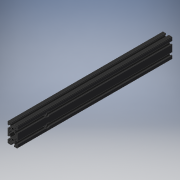
# Autodesk Inventor part: HFS5-2040-320-TPW-Z5-YA62.5
Saved by Autodesk Inventor 2019 (Build 230136000, 136)
## iProperties
Created: 2022-12-16
Part Number: HFS5-2040-320-TPW-Z5-YA62.5
Material: Generic
Catalog Web Link: www.cadenas.de
Description: NFS5-2040, NFSB5-2040, HFS5-2040, HFSB5-2040, CAF5-2040, NFSF5-2040, HFSF5-2040, HFSY5-2040-Aluminum Frames -5 Series-2Row Groove 20x40 mm Square -Specified Length
Vendor: MISUMI
Document SubType Name: Modeling
Designer: psAdmin
Manufacturer: MISUMI
Mass: 103.283 g
Surface Area: 1011.21 cm^2
Volume: 103.283 cm^3
Density: 1 g/cm^3
Appearance: PSOLRGB-175-175-175
Category: PARTsolutions
Company: MISUMI
Title: HFS5-2040-320-TPW-Z5-YA62.5
Author: Cadenas PARTsolutions
Comments: Aluminum Frames -5 Series-2Row Groove 20x40 mm Square -Specified Length
PSOL_IDENT_0: {$CADENAS_DATA/23d-libs/misumi/metric/38_al_extrusions_blackets/5/hfs5_2040.prj},655 {VTYP=3D},{NB=H
PSOL_IDENT_1: FS5-2040-320-TPW-Z5-YA62.5},{LINA=HFS5-2040-320-TPW-Z5-YA62.5},{NN=NFS5-2040, NFSB5-2040, HFS5-2040,
PSOL_IDENT_2: HFSB5-2040, CAF5-2040, NFSF5-2040, HFSF5-2040, HFSY5-2040},{DATE=23.09.2021 05:44:57},{GEOMDATE=23.
PSOL_IDENT_3: 09.2021 02:57:03},{VERSION=},{LINEID=150},{WBVAR=L,ALT1,ALT2,ALT4,ALT5,CP5,DL5,DR5,ALT6,ALT9,ALT10,A
PSOL_IDENT_4: LT11,HP6,NHL6,DL6,NHR6,DR6,ALT7,ALT8,NH9,AH,BH,CH,DH,EH,NH10,AV,BV,CV,DV,EV,NH11,AP,BP,CP,DP,EP,ALT1
PSOL_IDENT_5: 2,ALT13,Z,NH12,XA,XB,XC,XD,XE,NH13,YA,YB,YC,YD,YE,ALT16,HP16,DL16,DR16,ALT17,HQ17,JLP,ALT18,HQ18,KLP
PSOL_IDENT_6: ,ALT20},{WBNUMERIC=L,NH9,AH,BH,CH,DH,EH,NH10,AV,BV,CV,DV,EV,NH11,AP,BP,CP,DP,EP,NH12,XA,XB,XC,XD,XE,
PSOL_IDENT_7: NH13,YA,YB,YC,YD,YE,HQ17,JLP,HQ18,KLP}  {NB=HFS5-2040-320-TPW-Z5-YA62.5},{LINA=HFS5-2040-320-TPW-Z5-
PSOL_IDENT_8: YA62.5},{KT=DUMMY},{PN=HFS5-2040-320-TPW-Z5-YA62.5},{TPS=HFS5-2040},{MAT=A6N01SS-T5 Aluminum Alloy},
PSOL_IDENT_9: {ST=Clear Anodize},{FRMW=20},{FRMH=40},{FRD=4.2},{L=320},{MASS=0.88},{SA=324},{LX=1.358x10^4},{LY=5.
PSOL_IDENT_10: 13x10^4},{ALT1=TPW},{M1=5},{DPL1=15},{DPR1=15},{ALT1PN=-TPW},{ALT2=},{ALT2ALG= '','Not applicable' }
PSOL_IDENT_11: ,{M2=0},{DP2=0},{ALT2PN=},{ALT4=},{ALT4ALG= '', 'w/o SC (High Precision Cut)', 'SC', 'with SC (High
PSOL_IDENT_12: Precision Cut)' },{ALT4PN=},{ALT5=},{ALT5ALG= '','w/o 45 Degree Cut','1','with 45 Degree Cut' },{CP5=
PSOL_IDENT_13: },{CP5ALG= '','N/A' },{DL5=},{DL5ALG= '','N/A' },{DR5=},{DR5ALG= '','N/A' },{FRMLALT5=0},{FRMRALT5=0
PSOL_IDENT_14: },{ALT5PN=},{ALT6=},{ALT6ALG= '','w/o Fastening Location Wrench Access Hole Alterations','1','with F
PSOL_IDENT_15: astening Location Wrench Access Hole Alterations' },{ALT9=},{ALT9ALG= '','w/o Location Specified Wre
PSOL_IDENT_16: nch Access Hole Alteratons (Horizontal)','1','with Location Specified Wrench Access Hole Alteratons
PSOL_IDENT_17: (Horizontal)' },{ALT10=},{ALT10ALG= '','w/o Location Specified Wrench Access Hole Alteratons (Vertic
PSOL_IDENT_18: al)','1','with Location Specified Wrench Access Hole Alteratons (Vertical)' },{ALT11=},{ALT11ALG= ''
PSOL_IDENT_19: ,'w/o Location Specified Wrench Access Hole Alteratons (Crisscross)','1','with Location Specified Wr
PSOL_IDENT_20: ench Access Hole Alteratons (Crisscross)' },{HP6=},{HP6ALG= '','N/A' },{NHL6=},{NHL6ALG= '','N/A' },
PSOL_IDENT_21: {DL6=},{DL6ALG= '','N/A' },{NHR6=},{NHR6ALG= '','N/A' },{DR6=},{DR6ALG= '','N/A' },{HL6=0},{HL6D=0},
PSOL_IDENT_22: {HR6=0},{HR6D=0},{J6=0},{J6D=0},{K6=0},{K6D=0},{DD6=0.00},{DD6ALG=0},{ALT7=},{ALT7ALG= '','N/A' },{A
PSOL_IDENT_23: LT8=},{ALT8ALG= '','N/A' },{ALT678PN=},{NH9=0},{NH9MAX=5},{NH9ALG=[0]},{AH=0.0},{AHMIN=7},{AHMAX=315
PSOL_IDENT_24: },{AHALG=[0]},{BH=0.0},{BHMIN=2},{BHMAX=317},{BHALG=[0]},{CH=0.0},{CHMIN=2},{CHMAX=319},{CHALG=[0]},
PSOL_IDENT_25: {DH=0.0},{DHMIN=2},{DHMAX=321},{DHALG=[0]},{EH=0.0},{EHMIN=2},{EHMAX=313},{EHALG=[0]},{NH10=0},{NH10
PSOL_IDENT_26: MAX=5},{NH10ALG=[0]},{AV=0.0},{AVMIN=7},{AVMAX=315},{AVALG=[0]},{BV=0.0},{BVMIN=2},{BVMAX=317},{BVAL
PSOL_IDENT_27: G=[0]},{CV=0.0},{CVMIN=2},{CVMAX=319},{CVALG=[0]},{DV=0.0},{DVMIN=2},{DVMAX=321},{DVALG=[0]},{EV=0.0
PSOL_IDENT_28: },{EVMIN=2},{EVMAX=313},{EVALG=[0]},{NH11=0},{NH11MAX=5},{NH11ALG=[0]},{AP=0.0},{APMIN=7},{APMAX=315
PSOL_IDENT_29: },{APALG=[0]},{BP=0.0},{BPMIN=2},{BPMAX=317},{BPALG=[0]},{CP=0.0},{CPMIN=2},{CPMAX=319},{CPALG=[0]},
PSOL_IDENT_30: {DP=0.0},{DPMIN=2},{DPMAX=321},{DPALG=[0]},{EP=0.0},{EPMIN=2},{EPMAX=313},{EPALG=[0]},{ALT9PN=},{ALT
PSOL_IDENT_31: 10PN=},{ALT11PN=},{ALT91011PN=},{ALT12=},{ALT12ALG= '','w/o Counterbore Hole in Specified Position (
PSOL_IDENT_32: Vertical)','1','with Counterbore Hole in Specified Position (Vertical)' },{ALT13=1},{ALT13ALG= '','w
PSOL_IDENT_33: /o Counterbore Hole in Specified Position (Horizontal)','1','with Counterbore Hole in Specified Posi
PSOL_IDENT_34: tion (Horizontal)' },{Z=5},{ZALG='5','5','6','6'},{DD12=5.5},{DD112=9.5},{NH12=0},{NH12MAX=5},{NH12A
PSOL_IDENT_35: LG=[0]},{XA=0.0},{XAMIN=7},{XAMAX=324.5},{XAALG=[0]},{XB=0.0},{XBMIN=11.5},{XBMAX=336},{XBALG=[0]},{
PSOL_IDENT_36: XC=0.0},{XCMIN=11.5},{XCMAX=347.5},{XCALG=[0]},{XD=0.0},{XDMIN=11.5},{XDMAX=359},{XDALG=[0]},{XE=0.0
PSOL_IDENT_37: },{XEMIN=11.5},{XEMAX=313},{XEALG=[0]},{NH13=1},{NH13MAX=5},{NH13ALG=[1:5/1]},{YA=62.5},{YAMIN=7},{Y
PSOL_IDENT_38: AMAX=313},{YAALG=[7:313/0.5]},{YB=0.0},{YBMIN=74},{YBMAX=324.5},{YBALG=[0]},{YC=0.0},{YCMIN=11.5},{Y
PSOL_IDENT_39: CMAX=336},{YCALG=[0]},{YD=0.0},{YDMIN=11.5},{YDMAX=347.5},{YDALG=[0]},{YE=0.0},{YEMIN=11.5},{YEMAX=3
PSOL_IDENT_40: 13},{YEALG=[0]},{ALT12PN=},{ALT13PN=-YA62.5},{ALT1213PN=-Z5-YA62.5},{ALT16=},{ALT16ALG= '','w/o M Ty
PSOL_IDENT_41: pe Hole Alteration','1','with M Type Hole Alteration' },{HP16=},{HP16ALG= '','N/A' },{DL16=},{DL16AL
PSOL_IDENT_42: G= '','N/A' },{DR16=},{DR16ALG= '','N/A' },{H116=0},{D16=0.0},{ALT16PN=},{ALT17=},{ALT17ALG= '','w/o
PSOL_IDENT_43: L Type Hole Alteration (Top)','1','with L Type Hole Alteration (Top)' },{HQ17=0},{HQ17ALG=0},{JLP=0
PSOL_IDENT_44: },{JLPMIN=4.9},{JLPMAX=0},{JLPALG=[0]},{L17=0},{D17=0.0},{ALT18=},{ALT18ALG= '','w/o L Type Hole Alt
PSOL_IDENT_45: eration (Bottom)','1','with L Type Hole Alteration (Bottom)' },{HQ18=0},{HQ18ALG=0},{KLP=0},{KLPMIN=
PSOL_IDENT_46: 4.9},{KLPMAX=0},{KLPALG=[0]},{L18=0},{D18=0.0},{ALT1718PN=},{ALT20=},{ALT20PN=},{ERRORALT01=OK},{ERR
PSOL_IDENT_47: ORALT02=OK},{ERRORALT05=OK},{ERRORALT06091=OK},{ERRORALT06092=OK},{ERRORALT06093=OK},{ERRORALT06094=
PSOL_IDENT_48: OK},{ERRORALT06101=OK},{ERRORALT06102=OK},{ERRORALT06103=OK},{ERRORALT06104=OK},{ERRORALT06111=OK},{
PSOL_IDENT_49: ERRORALT06112=OK},{ERRORALT06113=OK},{ERRORALT06114=OK},{ERRORALT06121=OK},{ERRORALT06122=OK},{ERROR
PSOL_IDENT_50: ALT06123=OK},{ERRORALT06124=OK},{ERRORALT06131=OK},{ERRORALT06132=OK},{ERRORALT06133=OK},{ERRORALT06
PSOL_IDENT_51: 134=OK},{ERRORALT0616=OK},{ERRORALT06171=OK},{ERRORALT06172=OK},{ERRORALT06173=OK},{ERRORALT06181=OK
PSOL_IDENT_52: },{ERRORALT06182=OK},{ERRORALT06183=OK},{ERRORALT0911=OK},{ERRORALT0913=OK},{ERRORALT0916=OK},{ERROR
PSOL_IDENT_53: ALT0917=OK},{ERRORALT0918=OK},{ERRORALT1011=OK},{ERRORALT1012=OK},{ERRORALT1016=OK},{ERRORALT1017=OK
PSOL_IDENT_54: },{ERRORALT1018=OK},{ERRORALT1112=OK},{ERRORALT1113=OK},{ERRORALT1116=OK},{ERRORALT1117=OK},{ERRORAL
PSOL_IDENT_55: T1118=OK},{ERRORALT1216=OK},{ERRORALT1217=OK},{ERRORALT1218=OK},{ERRORALT1316=OK},{ERRORALT1317=OK},
PSOL_IDENT_56: {ERRORALT1318=OK},{ERRORALT1617=OK},{ERRORALT1618=OK},{ERRORPN=},{TFW=0},{COLOR=}
NB: HFS5-2040-320-TPW-Z5-YA62.5
NN: NFS5-2040, NFSB5-2040, HFS5-2040, HFSB5-2040, CAF5-2040, NFSF5-2040, HFSF5-2040, HFSY5-2040
NT: Aluminum Frames -5 Series-2Row Groove 20x40 mm Square -Specified Length
NBSYN: $PN.
LINA: HFS5-2040-320-TPW-Z5-YA62.5
CATALOG: Misumi
PN: HFS5-2040-320-TPW-Z5-YA62.5
TPS: HFS5-2040
MAT: A6N01SS-T5 Aluminum Alloy
ST: Clear Anodize
L: 320
MASS: 0.88
SA: 324
LX: 1.358x10^4
LY: 5.13x10^4
ALT1: with TPW (Tapping on Both Ends)
M1: 5
DPL1: 15
DPR1: 15
ALT2: Not applicable
M2: 0
DP2: 0
ALT4: w/o SC (High Precision Cut)
ALT5: w/o 45 Degree Cut
CP5: N/A
DL5: N/A
DR5: N/A
ALT6: w/o Fastening Location Wrench Access Hole Alterations
ALT9: w/o Location Specified Wrench Access Hole Alteratons (Horizontal)
ALT10: w/o Location Specified Wrench Access Hole Alteratons (Vertical)
ALT11: w/o Location Specified Wrench Access Hole Alteratons (Crisscross)
HP6: N/A
NHL6: N/A
DL6: N/A
NHR6: N/A
DR6: N/A
HL6D: 0
HR6D: 0
J6D: 0
K6D: 0
DD6: 0
ALT7: N/A
ALT8: N/A
NH9: 0
AH: 0
BH: 0
CH: 0
DH: 0
EH: 0
NH10: 0
AV: 0
BV: 0
CV: 0
DV: 0
EV: 0
NH11: 0
AP: 0
BP: 0
CP: 0
DP: 0
EP: 0
ALT12: w/o Counterbore Hole in Specified Position (Vertical)
ALT13: with Counterbore Hole in Specified Position (Horizontal)
Z: 5
DD12: 5.5
DD112: 9.5
NH12: 0
XA: 0
XB: 0
XC: 0
XD: 0
XE: 0
NH13: 1
YA: 62.5
YB: 0
YC: 0
YD: 0
YE: 0
ALT16: w/o M Type Hole Alteration
HP16: N/A
DL16: N/A
DR16: N/A
H116: 0
D16: 0
ALT17: w/o L Type Hole Alteration (Top)
HQ17: 0
JLP: 0
D17: 0
ALT18: w/o L Type Hole Alteration (Bottom)
HQ18: 0
KLP: 0
D18: 0
ALT20: w/o CW (End Face C Chamfering)
SUPPLIER: MISUMI
ARTICLENO: HFS5-2040-320-TPW-Z5-YA62.5
BOMINFO: HFS5-2040-320-TPW-Z5-YA62.5
CREATOR: CADENAS GmbH
Autodesk Inventor part; units mm, degrees
ref_plane "YZ Plane" through (0, 0, 0) normal (1, 0, 0) x (0, 1, 0)
ref_plane "XZ Plane" through (0, 0, 0) normal (0, 1, 0) x (-1, 0, 0)
ref_plane "XY Plane" through (0, 0, 0) normal (0, 0, 1) x (1, 0, 0)
sketch "Sketch_1" plane through (0, 0, 0) normal (0, 0, 1) x (1, 0, 0)
  line L0 (-10, -7) -> (-8, -7)
  line L1 (-8, -7) -> (-8, -4)
  line L2 (-8, -4) -> (-7.0607, -4)
  line L3 (-7.0607, -4) -> (-4, -7.0607)
  line L4 (-4, -7.0607) -> (-4, -9.4804)
  line L5 (-4, -9.4804) -> (-3.7, -10)
  line L6 (-3.7, -10) -> (-4, -10.5196)
  line L7 (-4, -10.5196) -> (-4, -12.9393)
  line L8 (-4, -12.9393) -> (-7.0607, -16)
  line L9 (-7.0607, -16) -> (-8, -16)
  line L10 (-8, -16) -> (-8, -13)
  line L11 (-8, -13) -> (-10, -13)
  line L12 (-10, -13) -> (-10, -19)
  arc A0 (-10, -19) -> (-9, -20) centre (-9, -19) ccw
  line L13 (-9, -20) -> (-3, -20)
  line L14 (-3, -20) -> (-3, -18)
  line L15 (-3, -18) -> (-6, -18)
  line L16 (-6, -18) -> (-6, -17.0607)
  line L17 (-6, -17.0607) -> (-2.9393, -14)
  line L18 (-2.9393, -14) -> (-0.5196, -14)
  line L19 (-0.5196, -14) -> (0, -13.7)
  line L20 (0, -13.7) -> (0.5196, -14)
  line L21 (0.5196, -14) -> (2.9393, -14)
  line L22 (2.9393, -14) -> (6, -17.0607)
  line L23 (6, -17.0607) -> (6, -18)
  line L24 (6, -18) -> (3, -18)
  line L25 (3, -18) -> (3, -20)
  line L26 (3, -20) -> (9, -20)
  arc A1 (9, -20) -> (10, -19) centre (9, -19) ccw
  line L27 (10, -19) -> (10, -13)
  line L28 (10, -13) -> (8, -13)
  line L29 (8, -13) -> (8, -16)
  line L30 (8, -16) -> (7.0607, -16)
  line L31 (7.0607, -16) -> (4, -12.9393)
  line L32 (4, -12.9393) -> (4, -10.5196)
  line L33 (4, -10.5196) -> (3.7, -10)
  line L34 (3.7, -10) -> (4, -9.4804)
  line L35 (4, -9.4804) -> (4, -7.0607)
  line L36 (4, -7.0607) -> (7.0607, -4)
  line L37 (7.0607, -4) -> (8, -4)
  line L38 (8, -4) -> (8, -7)
  line L39 (8, -7) -> (10, -7)
  line L40 (10, -7) -> (10, 7)
  line L41 (10, 7) -> (8, 7)
  line L42 (8, 7) -> (8, 4)
  line L43 (8, 4) -> (7.0607, 4)
  line L44 (7.0607, 4) -> (4, 7.0607)
  line L45 (4, 7.0607) -> (4, 9.4804)
  line L46 (4, 9.4804) -> (3.7, 10)
  line L47 (3.7, 10) -> (4, 10.5196)
  line L48 (4, 10.5196) -> (4, 12.9393)
  line L49 (4, 12.9393) -> (7.0607, 16)
  line L50 (7.0607, 16) -> (8, 16)
  line L51 (8, 16) -> (8, 13)
  line L52 (8, 13) -> (10, 13)
  line L53 (10, 13) -> (10, 19)
  arc A2 (10, 19) -> (9, 20) centre (9, 19) ccw
  line L54 (9, 20) -> (3, 20)
  line L55 (3, 20) -> (3, 18)
  line L56 (3, 18) -> (6, 18)
  line L57 (6, 18) -> (6, 17.0607)
  line L58 (6, 17.0607) -> (2.9393, 14)
  line L59 (2.9393, 14) -> (0.5196, 14)
  line L60 (0.5196, 14) -> (0, 13.7)
  line L61 (0, 13.7) -> (-0.5196, 14)
  line L62 (-0.5196, 14) -> (-2.9393, 14)
  line L63 (-2.9393, 14) -> (-6, 17.0607)
  line L64 (-6, 17.0607) -> (-6, 18)
  line L65 (-6, 18) -> (-3, 18)
  line L66 (-3, 18) -> (-3, 20)
  line L67 (-3, 20) -> (-9, 20)
  arc A3 (-9, 20) -> (-10, 19) centre (-9, 19) ccw
  line L68 (-10, 19) -> (-10, 13)
  line L69 (-10, 13) -> (-8, 13)
  line L70 (-8, 13) -> (-8, 16)
  line L71 (-8, 16) -> (-7.0607, 16)
  line L72 (-7.0607, 16) -> (-4, 12.9393)
  line L73 (-4, 12.9393) -> (-4, 10.5196)
  line L74 (-4, 10.5196) -> (-3.7, 10)
  line L75 (-3.7, 10) -> (-4, 9.4804)
  line L76 (-4, 9.4804) -> (-4, 7.0607)
  line L77 (-4, 7.0607) -> (-7.0607, 4)
  line L78 (-7.0607, 4) -> (-8, 4)
  line L79 (-8, 4) -> (-8, 7)
  line L80 (-8, 7) -> (-10, 7)
  line L81 (-10, 7) -> (-10, -7)
  line L82 (-8, 1.7) -> (-8, -1.7)
  arc A4 (-8, -1.7) -> (-7.7, -2) centre (-7.7, -1.7) ccw
  line L83 (-7.7, -2) -> (-7.0636, -2)
  arc A5 (-6.8515, -2.0879) -> (-7.0636, -2) centre (-7.0636, -2.3) ccw
  line L84 (-6.8515, -2.0879) -> (-2.9393, -6)
  line L85 (-2.9393, -6) -> (2.9393, -6)
  line L86 (2.9393, -6) -> (6.8515, -2.0879)
  arc A6 (7.0636, -2) -> (6.8515, -2.0879) centre (7.0636, -2.3) ccw
  line L87 (7.0636, -2) -> (7.7, -2)
  arc A7 (7.7, -2) -> (8, -1.7) centre (7.7, -1.7) ccw
  line L88 (8, -1.7) -> (8, 1.7)
  arc A8 (8, 1.7) -> (7.7, 2) centre (7.7, 1.7) ccw
  line L89 (7.7, 2) -> (7.0636, 2)
  arc A9 (6.8515, 2.0879) -> (7.0636, 2) centre (7.0636, 2.3) ccw
  line L90 (6.8515, 2.0879) -> (2.9393, 6)
  line L91 (2.9393, 6) -> (-2.9393, 6)
  line L92 (-2.9393, 6) -> (-6.8515, 2.0879)
  arc A10 (-7.0636, 2) -> (-6.8515, 2.0879) centre (-7.0636, 2.3) ccw
  line L93 (-7.0636, 2) -> (-7.7, 2)
  arc A11 (-7.7, 2) -> (-8, 1.7) centre (-7.7, 1.7) ccw
  constraints: 188 end point, 24 point on circle, 12 centre point
extrude "Extrusion1" add sketch "Sketch_1" against normal blind 320
sketch "Sketch2" plane through (0, 0, 0) normal (0, 0, 1) x (1, 0, 0)
  point P0 (0, 10)
hole "Hole1" at (0, 10, 0) direction (0, 0, -1) diameter 4.134 depth 15 countersink diameter 5 countersink angle 90 thread size "M5x0.8" class "6H" standard "ISO Metric profile"
pattern_linear "Rectangular Pattern1" count 2 spacing 20 along (0, -1, 0) of "Hole1"
sketch "Sketch3" plane through (0, 0, -320) normal (0, 0, -1) x (-1, 0, 0)
  point P0 (0, 10)
hole "Hole2" at (0, 10, -320) direction (0, 0, 1) diameter 4.134 depth 15 countersink diameter 5 countersink angle 90 thread size "M5x0.8" class "6H" standard "ISO Metric profile"
pattern_linear "Rectangular Pattern2" count 2 spacing 20 along (0, -1, 0) of "Hole2"
sketch "Sketch4" plane through (0, 10, -305) normal (0, 0, -1) x (-1, 0, 0)
  point P0 (0, 0)
hole "Hole3" at (0, 10, -305) direction (0, 0, 1) diameter 4.2 depth 290
pattern_linear "Rectangular Pattern3" count 2 spacing 20 along (0, -1, 0) of "Hole3"
sketch "Sketch_50" plane through (0, 10, 0) normal (0, 1, 0) x (1, 0, 0)
  line L0 (10, 62.5) -> (-10, 62.5)
  line L1 (-10, 62.5) -> (-10, 65.25)
  line L2 (-10, 65.25) -> (4, 65.25)
  line L3 (4, 65.25) -> (4, 67.25)
  line L4 (4, 67.25) -> (10, 67.25)
  line L5 (10, 67.25) -> (10, 62.5)
  line L6 (10, 62.5) -> (-10, 62.5)
  constraints: 14 end point
revolve "Revolution1" cut sketch "Sketch_50" angle 360 about axis through (10, 10, -62.5) along (1, 0, 0)
sketch "_p_______27_Sketch_50_0" plane through (0, -10, 0) normal (0, 1, 0) x (1, 0, 0)
  line L0 (10, 62.5) -> (-10, 62.5)
  line L1 (-10, 62.5) -> (-10, 65.25)
  line L2 (-10, 65.25) -> (4, 65.25)
  line L3 (4, 65.25) -> (4, 67.25)
  line L4 (4, 67.25) -> (10, 67.25)
  line L5 (10, 67.25) -> (10, 62.5)
  line L6 (10, 62.5) -> (-10, 62.5)
  constraints: 14 end point
revolve "Revolution2" cut sketch "_p_______27_Sketch_50_0" angle 360 about axis through (10, -10, -62.5) along (1, 0, 0)
ref_plane "C1_XY" through (0, 0, 0) normal (0, 0, 1) x (1, 0, 0)
ref_plane "C1_YZ" through (0, 0, 0) normal (1, 0, 0) x (0, 1, 0)
ref_plane "C1_ZX" through (0, 0, 0) normal (0, 1, 0) x (0, 0, 1)
body "Solid1"
